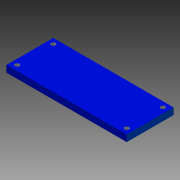
# Autodesk Inventor part: ライントレース
Saved by Autodesk Inventor 2015 (Build 190159000, 159)
## iProperties
Created: 2015-05-18
Part Number: ライントレース
Material: アセタール樹脂、白
Document SubType Name: Modeling
Designer: kenta
Density: 1.425 g/cm^3
Appearance: 滑らか - 白
Mass: 22.2145 g
Surface Area: 76.8672 cm^2
Volume: 15.5892 cm^3
Author: kenta
Autodesk Inventor part; units mm, degrees
ref_plane "YZ Plane" through (0, 0, 0) normal (1, 0, 0) x (0, 1, 0)
ref_plane "XZ Plane" through (0, 0, 0) normal (0, 1, 0) x (-1, 0, 0)
ref_plane "XY Plane" through (0, 0, 0) normal (0, 0, 1) x (1, 0, 0)
sketch "スケッチ1" plane through (0, 0, 0) normal (0, 0, 1) x (1, 0, 0)
  line L0 (-45, 17.5) -> (45, 17.5)
  line L1 (45, 17.5) -> (45, -17.5)
  line L2 (45, -17.5) -> (-45, -17.5)
  line L3 (-45, -17.5) -> (-45, 17.5)
  line L4 (-45, 17.5) -> (45, -17.5) construction
  line L5 (45, 17.5) -> (-45, -17.5) construction
  point P0 (0, 0)
  dimension "d0" = 90
  dimension "d1" = 35
  constraints: 12 end point, 2 midpoint, 2 parallel, 1 horizontal, 1 perpendicular
  measures "d0" distance of L1.end L2.end
  measures "d1" distance of L0.end L1.end
extrude "押し出し1" add sketch "スケッチ1" along normal blind 5
sketch "スケッチ3" plane through (0, 0, 5) normal (0, 0, 1) x (1, 0, 0)
  line L0 (-45, 17.5) -> (-45, -17.5) projected
  line L1 (45, 17.5) -> (-45, 17.5) projected
  line L2 (-45, -17.5) -> (45, -17.5) projected
  line L3 (45, -17.5) -> (45, 17.5) projected
  point P0 (0, 0)
  point P1 (-41, 13.5)
  point P2 (-41, -13.5)
  point P3 (41, 13.5)
  point P4 (41, -13.5)
  dimension "d15" = 4
  dimension "d16" = 4
  dimension "d17" = 4
  dimension "d18" = 4
  dimension "d19" = 4
  dimension "d20" = 4
  dimension "d21" = 4
  dimension "d29" = 82
  dimension "d31" = 4
  dimension "d32" = 27
  measures "d15" distance from line of L0 point (-41, 13.5)
  measures "d16" distance from line of point (-41, 13.5) L1
  measures "d17" distance from line of L0 point (-41, -13.5)
  measures "d18" distance from line of point (-41, -13.5) L2
  measures "d19" distance from line of L2 point (41, -13.5)
  measures "d20" distance from line of point (41, 13.5) L3
  measures "d21" distance from line of point (41, -13.5) L3
  measures "d29" distance of point (41, 13.5) point (-41, 13.5)
  measures "d31" distance from line of L1 point (41, 13.5)
  measures "d32" distance of point (41, -13.5) point (41, 13.5)
hole "穴2" at (-41, 13.5, 5) at (-41, -13.5, 5) at (41, 13.5, 5) at (41, -13.5, 5) direction (0, 0, -1) diameter 3.2 depth 8 tip angle 118
